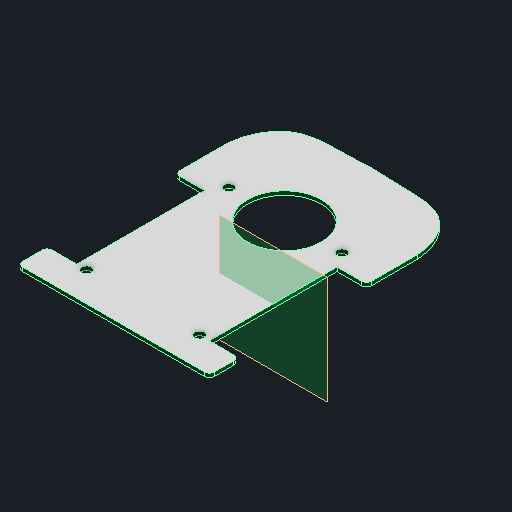
# Autodesk Inventor part: MainBoard
Saved by Autodesk Inventor 2023 (Build 270158000, 158)
## iProperties
Created: 2022-03-27
Part Number: MainBoard
Material: 一般
Document SubType Name: Modeling
Designer: neko2
Density: 1 g/cm^3
Appearance: 既定
Author: neko2
Autodesk Inventor part; units mm, degrees
ref_plane "YZ Plane" through (0, 0, 0) normal (1, 0, 0) x (0, 1, 0)
ref_plane "XZ Plane" through (0, 0, 0) normal (0, 1, 0) x (-1, 0, 0)
ref_plane "XY Plane" through (0, 0, 0) normal (0, 0, 1) x (1, 0, 0)
sketch "スケッチ1" plane through (0, 0, 0) normal (0, 1, 0) x (-1, 0, 0)
  line L0 (-13.5, 21) -> (-19.5, 21)
  line L1 (-19.5, 21) -> (-19.5, 0)
  line L2 (-19.5, 0) -> (19.5, 0)
  line L3 (19.5, 0) -> (19.5, 21)
  line L4 (19.5, 21) -> (13.5, 21)
  line L5 (13.5, 21) -> (13.5, 47)
  line L6 (13.5, 47) -> (19.5, 47)
  line L7 (19.5, 47) -> (19.5, 53)
  line L8 (19.5, 53) -> (-19.5, 53)
  line L9 (-19.5, 53) -> (-19.5, 47)
  line L10 (-19.5, 47) -> (-13.5, 47)
  line L11 (-13.5, 47) -> (-13.5, 21)
  point P0 (0, 0)
  point P1 (0, 0)
  dimension "d5" = 39
  dimension "d6" = 27
  dimension "d8" = 26
  dimension "d16" = 6
  dimension "d43" = 53
  dimension "d44" = 39
  constraints: 24 end point, 7 perpendicular, 2 collinear, 2 horizontal, 2 midpoint, 2 point on line, 2 vertical, 1 coincident, 1 horizontal alignment
  measures "d5" distance of L7.end L8.end
  measures "d6" distance between parallel lines of L11 L5
  measures "d8" distance of L10.end L0.start
  measures "d16" distance of L6.end L7.end
  measures "d43" distance between parallel lines of L2 L8
  measures "d44" distance between parallel lines of L3 L1
extrude "Body" add sketch "スケッチ1" along normal blind 0.8
fillet "フィレット1" radius 1 6 edges at (19.5, 0.4, 53) (19.5, 0.4, 47) (19.5, 0.4, 21) (-19.5, 0.4, 21) (-19.5, 0.4, 53) (-19.5, 0.4, 47)
sketch "スケッチ6" plane through (0, 0, 0) normal (0, -1, 0) x (1, 0, 0)
  circle A0 centre (0, 18.2) radius 7.5
  line L0 (19.5, 0) -> (-19.5, 0) projected
  circle A1 centre (0, 18.2) radius 10
  point P0 (0, 0)
  point P1 (0, 0)
  dimension "d27" = 15
  dimension "d28" = 20
  dimension "d31" = 18.2
  constraints: 2 centre point, 1 coincident, 1 midpoint, 1 vertical alignment
  measures "d27" diameter of A0
  measures "d28" diameter of A1
  measures "d31" distance from line of A0.centre L0
extrude "押し出し4" cut sketch "スケッチ6" against normal through all contours A0
sketch "スケッチ7" plane through (0, 0.8, 0) normal (0, 1, 0) x (1, 0, 0)
  spline S0 degree 5 poles (0, 0) (-0.3117, -0.0168) (-0.9317, -0.0488) (-1.8515, -0.0923) (-3.0577, -0.1409) (-4.5307, -0.1873) (-5.9672, -0.223) (-7.3645, -0.2562) (-8.7185, -0.3001) (-10.0237, -0.3761) (-11.2732, -0.5129) (-12.4592, -0.7408) (-13.5734, -1.0876) (-14.6076, -1.5729) (-15.5546, -2.2027) (-16.4082, -2.9673) (-17.1633, -3.8489) (-17.8162, -4.8254) (-18.3648, -5.8755) (-18.8088, -6.9843) (-19.1492, -8.1424) (-19.3399, -9.1044) (-19.4375, -9.8448) (-19.4825, -10.3469) (-19.5, -10.6) knots 0 0 0 0 0 0 0.05 0.1 0.15 0.2 0.25 0.3 0.35 0.4 0.45 0.5 0.55 0.6 0.65 0.7 0.75 0.8 0.85 0.9 0.95 1 1 1 1 1 1
  spline S1 degree 5 poles (19.5, -10.6) (19.4825, -10.3469) (19.4375, -9.8448) (19.3399, -9.1043) (19.1492, -8.1424) (18.8088, -6.9842) (18.3648, -5.8755) (17.8162, -4.8253) (17.1633, -3.8489) (16.4081, -2.9673) (15.5546, -2.2027) (14.6076, -1.5729) (13.5734, -1.0876) (12.4592, -0.7408) (11.2732, -0.5129) (10.0237, -0.3762) (8.7184, -0.3002) (7.3644, -0.2562) (5.9671, -0.2231) (4.5306, -0.1873) (3.0577, -0.141) (1.8515, -0.0923) (0.9316, -0.0489) (0.3116, -0.0169) (0, 0) knots -1 -1 -1 -1 -1 -1 -0.95 -0.9 -0.85 -0.8 -0.75 -0.7 -0.65 -0.6 -0.55 -0.5 -0.45 -0.4 -0.35 -0.3 -0.25 -0.2 -0.15 -0.1 -0.05 0 0 0 0 0 0
  line L0 (19.5, -10.6) -> (19.5, -53)
  line L1 (19.5, -53) -> (-19.5, -53)
  line L2 (-19.5, -53) -> (-19.5, -10.6)
  line L3 (-18.5, -53) -> (18.5, -53) projected
  line L4 (19.5, 0) -> (-19.5, 0) projected
  point P0 (0, -53)
  dimension "d40" = 53
  dimension "d45" = 39
  dimension "d47" = 10.6
  constraints: 6 end point, 2 midpoint, 2 perpendicular, 1 horizontal alignment, 1 vertical, 1 vertical alignment, 4 other
  measures "d40" distance from line of point (0, 0) L1
  measures "d45" distance between parallel lines of L2 L0
  measures "d47" vertical distance of point (0, 0) L2.end
extrude "押し出し5" cut sketch "スケッチ7" against normal through all keep common part
sketch "スケッチ9" plane through (0, 0, 0) normal (0, -1, 0) x (1, 0, 0)
  circle A0 centre (-11.5, 47) radius 1
  circle A1 centre (-11.5, 47) radius 1
  circle A2 centre (-11.5, 18) radius 1
  line L0 (0, 0) -> (0, 53)
  circle A3 centre (11.5, 47) radius 1
  circle A4 centre (11.5, 47) radius 1
  circle A5 centre (11.5, 18) radius 1
  line L1 (-18.5, 53) -> (18.5, 53) projected
  circle A6 centre (0, 18.2) radius 7.5 projected
  line L2 (19.5, 20) -> (19.5, 10.6) projected
  arc A7 (19.5, 20) -> (18.5, 21) centre (18.5, 20) ccw projected
  line L3 (13.5, 21) -> (18.5, 21) projected
  line L4 (13.5, 47) -> (13.5, 21) projected
  line L5 (18.5, 47) -> (13.5, 47) projected
  arc A8 (18.5, 47) -> (19.5, 48) centre (18.5, 48) ccw projected
  line L6 (19.5, 52) -> (19.5, 48) projected
  arc A9 (19.5, 52) -> (18.5, 53) centre (18.5, 52) ccw projected
  line L7 (-18.5, 53) -> (18.5, 53) projected
  arc A10 (-18.5, 53) -> (-19.5, 52) centre (-18.5, 52) ccw projected
  line L8 (-19.5, 48) -> (-19.5, 52) projected
  arc A11 (-19.5, 48) -> (-18.5, 47) centre (-18.5, 48) ccw projected
  line L9 (-13.5, 47) -> (-18.5, 47) projected
  line L10 (-13.5, 21) -> (-13.5, 47) projected
  line L11 (-18.5, 21) -> (-13.5, 21) projected
  arc A12 (-18.5, 21) -> (-19.5, 20) centre (-18.5, 20) ccw projected
  line L12 (-19.5, 10.6) -> (-19.5, 20) projected
  dimension "d52" = 2
  dimension "d53" = 29
  dimension "d55" = 2
  constraints: 6 centre point, 3 coincident, 3 symmetric about line, 2 end point, 2 equal radius, 1 horizontal alignment, 1 midpoint, 1 vertical, 1 vertical alignment, 5 other
  measures "d52" diameter of A2
  measures "d53" distance of A0.centre A2.centre
  measures "d55" distance from line of A0.centre L10
extrude "押し出し7" cut sketch "スケッチ9" against normal through all contours A0 | A2 | A3 | A5
ref_plane "作業平面1" through (13.5, 0, 34) normal (0, 0, -1) x (-1, 0, 0)
